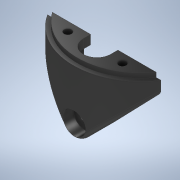
# Autodesk Inventor part: WheelBracketNut
Saved by Autodesk Inventor 2020 (Build 240168000, 168)
## iProperties
Created: 2019-05-28
Part Number: WheelBracketNut
Material: ABS Plastic
Document SubType Name: Modeling
Designer: Connor
Density: 1.06 g/cm^3
Appearance: Glossy - Black
Author: Connor
Autodesk Inventor part; units mm, degrees
ref_plane "YZ Plane" through (0, 0, 0) normal (1, 0, 0) x (0, 1, 0)
sketch "Sketch1" plane through (0, 0, 0) normal (0, 0, 1) x (1, 0, 0)
  line L0 (0, 0) -> (46.99, 0)
  line L1 (46.99, 0) -> (46.99, 44.45)
  line L2 (46.99, 44.45) -> (0, 44.45)
  line L3 (0, 44.45) -> (0, 0)
  line L4 (0, 44.45) -> (44.196, 44.45)
  line L5 (44.196, 44.45) -> (44.196, 47.6504)
  line L6 (44.196, 47.6504) -> (0, 47.6504)
  line L7 (0, 47.6504) -> (0, 44.45)
  circle A0 centre (0, 9.525) radius 9.525
  circle A1 centre (0, 9.525) radius 3.175
  line L8 (46.99, 44.45) -> (6.8499, 2.9065)
  line L9 (0, 0) -> (-46.99, 0)
  line L10 (-46.99, 0) -> (-46.99, 44.45)
  line L11 (-46.99, 44.45) -> (0, 44.45)
  line L12 (0, 44.45) -> (0, 0)
  line L13 (-46.99, 44.45) -> (-6.8499, 2.9065)
  dimension "d2" = 44.196
  dimension "d3" = 3.2004
  dimension "d5" = 6.35
  dimension "d7" = 6.35
  dimension "d85" = 34.925
  dimension "d126" = 46.99
  constraints: 28 end point, 6 parallel, 3 horizontal, 3 perpendicular, 3 point on circle, 2 centre point, 2 equal length, 2 tangent, 1 coincident, 1 point on line
  measures "d2" distance of L6.end L5.end
  measures "d3" distance of L5.end L4.end
  measures "d5" diameter of A1
  measures "d7" radial gap between concentric circles of A1 A0
  measures "d85" distance from line of A0.centre L11
  measures "d126" distance between parallel lines of L7 L1
revolve "Revolution1" add sketch "Sketch1" angle 180 about axis through (0, 44.45, 0) along (0, -1, 0) picked at (7.3287, 10.2315) picked at (0.9535, 9.9842) contours A0 L8 L1 L0 | L3 A1 A0 | L3 A1 | A0 L3 L2 L8 | L2 L7 L6 L5
sketch "Sketch2" plane through (0, 0, 0) normal (1, 0, 0) x (0, 1, 0)
  line L0 (0, 0) -> (44.45, 0) projected
  line L1 (47.6504, 44.196) -> (47.6504, 0) projected
  line L2 (0, 0) -> (47.6504, 0)
  line L3 (47.6504, 0) -> (47.6504, 25.4)
  line L4 (47.6504, 25.4) -> (0, 25.4)
  line L5 (0, 25.4) -> (0, 0)
  point P0 (44.45, 0)
  dimension "d10" = 25.4
  constraints: 8 end point, 2 parallel, 1 horizontal, 1 perpendicular, 1 point on line
  measures "d10" distance between parallel lines of L0 L4
extrude "Extrusion1" cut sketch "Sketch2" along normal through all both and the other way through all
extrude "Extrusion3" cut sketch "Sketch1" along normal through all contours A0 L8 L1 L0 | L9 L10 L13 A0
ref_plane "Work Plane3" through (0, 0, 0) normal (0, 1, 0) x (-1, 0, 0)
sketch "Sketch9" plane through (0, 0, 0) normal (0, 1, 0) x (-1, 0, 0)
  line L0 (-19.05, 31.75) -> (0, 0) construction
  line L1 (0, 0) -> (19.05, 31.75) construction
  dimension "d46" = 31.75
  dimension "d47" = 38.1
  constraints: 4 end point, 1 equal length, 1 horizontal alignment
  measures "d46" vertical distance of L0.end L0.start
  measures "d47" distance of L1.end L0.start
hole "Hole3" at (19.05, 0, 31.75) at (-19.05, 0, 31.75) direction (0, 1, 0) diameter 5.207 end through all counterbore diameter 8.7313 counterbore depth 25.4
ref_plane "Work Plane6" through (0, 22.225, 46.99) normal (0, 0, -1) x (-1, 0, 0)
sketch "Sketch19" plane through (0, 22.225, 46.99) normal (0, 0, -1) x (-1, 0, 0)
  circle A0 centre (0, -12.7) radius 9.525 construction
  arc A1 (-6.8499, -19.3185) -> (6.8499, -19.3185) centre (0, -12.7) ccw projected
  point P0 (0, -22.225)
  constraints: 2 concentric, 1 centre point, 1 coincident
hole "Hole5" at (0, 9.525, 46.99) direction (0, 0, -1) diameter 6.7564 end through all counterbore diameter 15.875 counterbore depth 7.9502
sketch "Sketch20" plane through (0, 0, 0) normal (1, 0, 0) x (0, 1, 0)
  line L0 (47.6504, 30.48) -> (22.225, 30.48)
  line L1 (22.225, 30.48) -> (22.225, 21.2094)
  line L2 (22.225, 21.2094) -> (30.3217, 16.1925)
  line L3 (38.919, 16.1925) -> (41.3004, 20.955)
  line L4 (41.3004, 20.955) -> (47.6504, 20.955)
  line L5 (47.6504, 20.955) -> (47.6504, 30.48)
  line L6 (12.9032, 25.4) -> (6.1468, 25.4) projected
  line L7 (30.3217, 16.1925) -> (38.919, 16.1925)
  line L8 (47.6504, 44.196) -> (47.6504, 25.4) projected
  point P0 (0, 0)
  point P1 (9.525, 25.4)
  dimension "d93" = 9.525
  dimension "d95" = 9.525
  dimension "d99" = 30.48
  dimension "d111" = 12.7
  dimension "d112" = 31.783
  dimension "d113" = 63.433
  dimension "d114" = 14.2875
  dimension "d115" = 6.35
  constraints: 14 end point, 2 horizontal, 2 perpendicular, 1 collinear, 1 midpoint, 1 parallel
  measures "d93" distance of L4.end L0.start
  measures "d95" distance of L2.end L1.end
  measures "d99" distance from line of point (0, 0) L0
  measures "d111" distance from line of point (9.525, 25.4) L1
  measures "d112" angle of L7 L2
  measures "d113" angle of L7 L3
  measures "d114" distance between parallel lines of L7 L0
  measures "d115" distance of L3.end L4.end
revolve "Revolution2" cut sketch "Sketch20" angle 360 about axis through (0, 47.6504, 30.48) along (0, -1, 0)
sketch "Sketch21" plane through (39.5335, 44.45, 25.4) normal (0, 0, -1) x (-1, 0, 0)
  line L0 (30.0085, -3.1496) -> (30.0085, 3.2004) projected
  line L1 (25.246, -5.531) -> (30.0085, -3.1496) projected
  line L2 (25.246, -14.1283) -> (25.246, -5.531) projected
  line L3 (30.2629, -22.225) -> (25.246, -14.1283) projected
  line L4 (48.8041, -22.225) -> (30.2629, -22.225) projected
  line L5 (48.8041, -22.225) -> (53.821, -14.1283) projected
  line L6 (53.821, -14.1283) -> (53.821, -5.531) projected
  line L7 (53.821, -5.531) -> (49.0585, -3.1496) projected
  line L8 (49.0585, -3.1496) -> (49.0585, 3.2004) projected
  line L9 (30.0085, 3.2004) -> (49.0585, 3.2004) projected
  line L10 (49.0585, -3.1496) -> (30.0085, -3.1496) projected
  point P0 (39.5335, -44.45)
  point P1 (47.2884, -22.225)
  point P2 (31.7787, -22.225)
  point P3 (31.4763, 3.2004)
  point P4 (47.5908, 3.2004)
  point P5 (47.5908, -3.1496)
  point P6 (31.4763, -3.1496)
extrude "Extrusion13" cut sketch "Sketch21" against normal blind 5.08
fillet "Fillet3" radius 3.175 4 edges at (3.9363, 0.8514, 46.8248) (-3.9246, 0.8461, 46.8258) (-25.4761, 22.1839, 39.4845) (25.4761, 22.1839, 39.4845)
fillet "Fillet1" radius 0.7937 2 edges at (19.05, 15.5331, 36.1156) (-19.05, 15.5331, 36.1156)
sketch "Sketch23" plane through (0, 22.225, 30.48) normal (0, 1, 0) x (1, 0, 0)
  circle A0 centre (0, 0) radius 6.477
  arc A1 (-9.2706, 0) -> (9.2706, 0) centre (0, 0) ccw projected
  point P0 (0, 30.48)
  dimension "d116" = 12.954
  constraints: 1 centre point, 1 concentric
  measures "d116" diameter of A0
hole "Hole6" at (0, 22.225, 30.48) direction (0, -1, 0) diameter 8.89 depth 6.35 counterbore diameter 12.954 counterbore depth 4.7752
body "Solid1"
